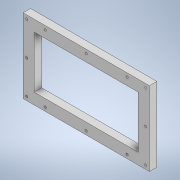
# Autodesk Inventor part: top
Saved by Autodesk Inventor 2022.2 (Build 262287030, 287C)
## iProperties
Created: 2022-01-28
Part Number: top
Material: Generic
Document SubType Name: Modeling
Designer: Tapendra
Density: 1 g/cm^3
Appearance: Default
Author: Tapendra
Autodesk Inventor part; units mm, degrees
ref_plane "YZ Plane" through (0, 0, 0) normal (1, 0, 0) x (0, 1, 0)
ref_plane "XZ Plane" through (0, 0, 0) normal (0, 1, 0) x (-1, 0, 0)
ref_plane "XY Plane" through (0, 0, 0) normal (0, 0, 1) x (1, 0, 0)
sketch "Sketch1" plane through (0, 0, 0) normal (0, 0, 1) x (1, 0, 0)
  line L0 (-85, 50) -> (85, 50)
  line L1 (85, 50) -> (85, -50)
  line L2 (85, -50) -> (-85, -50)
  line L3 (-85, -50) -> (-85, 50)
  line L4 (-85, 50) -> (85, -50) construction
  line L5 (85, 50) -> (-85, -50) construction
  point P0 (0, 0)
  dimension "d0" = 170
  dimension "d1" = 100
  constraints: 12 end point, 2 midpoint, 2 parallel, 1 horizontal, 1 perpendicular
  measures "d0" distance of L0.start L0.end
  measures "d1" distance of L0.end L1.end
extrude "Extrusion1" add sketch "Sketch1" along normal mid plane 10
sketch "Sketch2" plane through (0, 0, 5) normal (0, 0, 1) x (1, 0, 0)
  line L0 (-70, 35) -> (70, 35)
  line L1 (70, 35) -> (70, -35)
  line L2 (70, -35) -> (-70, -35)
  line L3 (-70, -35) -> (-70, 35)
  line L4 (-70, 35) -> (70, -35) construction
  line L5 (70, 35) -> (-70, -35) construction
  point P0 (0, 0)
  dimension "d4" = 140
  dimension "d5" = 70
  constraints: 12 end point, 2 midpoint, 2 parallel, 1 horizontal, 1 perpendicular
  measures "d4" distance of L0.start L0.end
  measures "d5" distance of L0.end L1.end
extrude "Extrusion2" cut sketch "Sketch2" against normal blind 10
sketch "Sketch3" plane through (0, 0, -5) normal (0, 0, -1) x (-1, 0, 0)
  line L0 (-85, -50) -> (85, -50) projected
  line L1 (-85, 50) -> (-85, -50) projected
  line L2 (-85, 50) -> (85, 50) projected
  point P0 (0, 0)
  point P1 (-25, -45)
  point P2 (25, -45)
  point P3 (25, 45)
  point P4 (-25, 45)
  point P5 (-80, 25)
  point P6 (-80, -25)
  point P7 (80, 25)
  point P8 (80, -25)
  dimension "d45" = 5
  dimension "d55" = 50
  dimension "d62" = 160
  dimension "d127" = 5
  dimension "d128" = 5
  dimension "d129" = 5
  dimension "d131" = 25
  constraints: 1 horizontal, 1 vertical, 3 other
  measures "d45" distance from line of L0 point (-25, -45)
  measures "d55" distance of point (-80, 25) point (-80, -25)
  measures "d62" distance of point (-80, 25) point (80, 25)
  measures "d127" distance from line of L0 point (25, -45)
  measures "d128" distance from line of L2 point (25, 45)
  measures "d129" distance from line of L2 point (-25, 45)
  measures "d131" distance from line of L0 point (-80, -25)
hole "Hole1" at (25, -45, -5) at (-25, -45, -5) at (-25, 45, -5) at (25, 45, -5) at (80, -25, -5) at (80, 25, -5) at (-80, -25, -5) at (-80, 25, -5) direction (0, 0, 1) diameter 3.175 depth 5
sketch "Sketch4" plane through (0, 0, 5) normal (0, 0, 1) x (1, 0, 0)
  line L0 (-85, 50) -> (-85, -50) projected
  line L1 (85, 50) -> (-85, 50) projected
  line L2 (-85, -50) -> (85, -50) projected
  line L3 (85, -50) -> (85, 50) projected
  point P0 (0, 0)
  point P1 (-80, 0)
  point P2 (-80, -45)
  point P3 (0, -45)
  point P4 (-55, -45)
  point P5 (55, -45)
  point P6 (80, -45)
  point P7 (80, 0)
  point P8 (-80, 45)
  point P9 (-55, 45)
  point P10 (55, 45)
  point P11 (0, 45)
  point P12 (80, 45)
  dimension "d3" = 0
  dimension "d72" = 50
  dimension "d73" = 5
  dimension "d74" = 5
  dimension "d75" = 85
  dimension "d78" = 25
  dimension "d80" = 5
  dimension "d81" = 5
  dimension "d82" = 25
  dimension "d85" = 160
  dimension "d115" = 5
  dimension "d116" = 5
  dimension "d117" = 5
  dimension "d120" = 90
  dimension "d125" = 45
  constraints: 1 horizontal, 1 vertical, 6 other
  measures "d72" distance from line of L1 point (-80, 0)
  measures "d73" distance from line of L0 point (-80, -45)
  measures "d74" distance from line of L2 point (-80, -45)
  measures "d75" distance from line of point (0, -45) L0
  measures "d78" distance of point (-55, -45) point (-80, -45)
  measures "d80" distance from line of L3 point (80, -45)
  measures "d81" distance from line of L2 point (80, -45)
  measures "d82" distance of point (55, -45) point (80, -45)
  measures "d85" distance of point (-80, 0) point (80, 0)
  measures "d115" distance from line of L2 point (-55, -45)
  measures "d116" distance from line of L2 point (0, -45)
  measures "d117" distance from line of L2 point (55, -45)
  measures "d120" distance of point (-80, -45) point (-80, 45)
  measures "d125" distance of point (80, 0) point (80, -45)
hole "Hole2" at (-80, 0, 5) at (-80, -45, 5) at (0, -45, 5) at (-55, -45, 5) at (55, -45, 5) at (80, -45, 5) at (80, 0, 5) at (80, 45, 5) at (55, 45, 5) at (0, 45, 5) at (-55, 45, 5) at (-80, 45, 5) direction (0, 0, -1) diameter 3 depth 5
body "Solid1"
